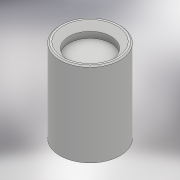
# Autodesk Inventor part: LENS
Saved by Autodesk Inventor 2017 (Build 210142000, 142)
## iProperties
Created: 2017-04-01
Part Number: LENS
Material: Generic
Document SubType Name: Modeling
Designer: Muchen
Density: 1 g/cm^3
Appearance: Default
Author: Muchen
Autodesk Inventor part; units mm, degrees
ref_plane "YZ Plane" through (0, 0, 0) normal (1, 0, 0) x (0, 1, 0)
ref_plane "XZ Plane" through (0, 0, 0) normal (0, 1, 0) x (-1, 0, 0)
ref_plane "XY Plane" through (0, 0, 0) normal (0, 0, 1) x (1, 0, 0)
sketch "Sketch1" plane through (0, 0, 0) normal (0, 0, 1) x (1, 0, 0)
  circle A0 centre (0, 0) radius 25
  circle A1 centre (0, 0) radius 17.5
  dimension "d0" = 35
  dimension "d1" = 50
  constraints: 2 centre point, 2 coincident
  measures "d0" diameter of A1
  measures "d1" diameter of A0
extrude "Extrusion1" add sketch "Sketch1" along normal mid plane 50 contours A1
extrude "Extrusion2" add sketch "Sketch1" along normal mid plane 70
chamfer "Chamfer1" distance 5 angle 45 1 edges at (-17.5, 0, 35)
chamfer "Chamfer2" distance 1 angle 45 1 edges at (-25, 0, 35)
chamfer "Chamfer3" distance 3 angle 45 2 edges at (-17.5, 0, -25) (-17.5, 0, -35)
body "Solid1"
